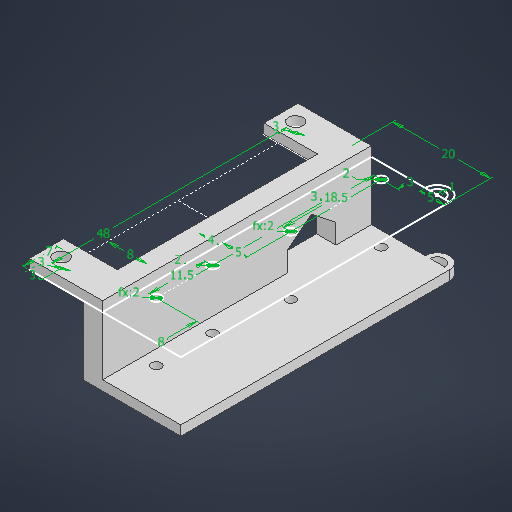
# Autodesk Inventor part: adcDAcmount
Saved by Autodesk Inventor 2025.1 (Build 291241000, 241)
## iProperties
Created: 2025-04-02
Part Number: adcDAcmount
Material: Generic
Document SubType Name: Modeling
Designer: jerem
Density: 1 g/cm^3
Appearance: Default
Author: jerem
## iProperties of the stored document adcDAcmount_3DPrint.ipt
Created: 2025-04-02
Part Number: adcDAcmount_3DPrint
Material: Generic
Document SubType Name: Modeling
Designer: jerem
Density: 1 g/cm^3
Appearance: Default
Author: jerem
Autodesk Inventor part; units mm, degrees
ref_plane "YZ Plane" through (0, 0, 0) normal (1, 0, 0) x (0, 1, 0)
ref_plane "XZ Plane" through (0, 0, 0) normal (0, 1, 0) x (-1, 0, 0)
ref_plane "XY Plane" through (0, 0, 0) normal (0, 0, 1) x (1, 0, 0)
sketch "Sketch1" plane through (0, 0, 0) normal (0, 1, 0) x (-1, 0, 0)
  line L0 (0, 0) -> (12, 0) construction
  line L1 (12, 24) -> (12, -24) construction
  circle A0 centre (12, 24) radius 1.5
  circle A1 centre (12, -24) radius 1.5
  line L2 (15, 27.5) -> (15, 20.5)
  line L3 (15, 20.5) -> (4, 20.5)
  line L4 (4, 20.5) -> (4, 0)
  line L5 (15, 27.5) -> (-16, 27.5)
  line L6 (4, 0) -> (12, 0) construction
  line L7 (15, -27.5) -> (15, -20.5)
  line L8 (15, -20.5) -> (4, -20.5)
  line L9 (4, -20.5) -> (4, 0)
  line L10 (15, -27.5) -> (-16, -27.5)
  line L11 (12, 24) -> (15, 24) construction
  line L12 (-16, 27.5) -> (-16, -27.5)
  line L13 (0, 27.5) -> (0, -27.5)
  line L14 (4, 20.5) -> (4, 27.5)
  line L15 (4, -20.5) -> (4, -27.5)
  circle A2 centre (-3, 8) radius 1
  circle A3 centre (-3, 19.5) radius 1
  line L16 (-3, 8) -> (-3, 19.5) construction
  circle A4 centre (-5, -24.5) radius 1
  circle A5 centre (-5, -6) radius 1
  line L17 (-5, -24.5) -> (-5, -6) construction
  arc A6 (-16, -27.5) -> (-11, -27.5) centre (-13.5, -27.5) ccw
  arc A7 (-15, -27.5) -> (-12, -27.5) centre (-13.5, -27.5) ccw
  point P0 (-12, -27.5)
  dimension "d0" = 3
  dimension "d1" = 3
  dimension "d2" = 3
  dimension "d3" = 7
  dimension "d4" = 48
  dimension "d5" = 8
  dimension "d7" = 4
  dimension "d12" = 20
  dimension "d13" = 2
  dimension "d14" = 2
  dimension "d15" = 11.5
  dimension "d16" = 3
  dimension "d17" = 2
  dimension "d18" = 2
  dimension "d19" = 18.5
  dimension "d20" = 5
  dimension "d23" = 8
  dimension "d24" = 3
  dimension "d27" = 5
  dimension "d28" = 1
  constraints: 36 end point, 8 centre point, 7 perpendicular, 6 point on line, 4 point on circle, 4 symmetric about line, 3 horizontal, 3 midpoint, 3 vertical, 2 coincident, 1 tangent
  measures "d0" diameter of A0
  measures "d1" diameter of A1
  measures "d2" distance of L11.start L11.end
  measures "d3" distance of L2.start L2.end
  measures "d4" distance of L1.start L1.end
  measures "d5" distance between parallel lines of L1 L4
  measures "d7" distance between parallel lines of L13 L4
  measures "d12" distance between parallel lines of L12 L15
  measures "d13" diameter of A2
  measures "d14" diameter of A3
  measures "d15" distance of L16.start L16.end
  measures "d16" distance between parallel lines of L13 L16
  measures "d17" diameter of A4
  measures "d18" diameter of A5
  measures "d19" distance of L17.start L17.end
  measures "d20" distance between parallel lines of L13 L17
  measures "d23" distance from line of L5 L16.end
  measures "d24" distance from line of L10 L17.start
  measures "d27" distance of L10.end A6.end
  measures "d28" radial gap between concentric circles of A6 A7
extrude "Extrusion1" add sketch "Sketch1" along normal blind 2 contours L2 L3 L14 L5 | L14 L4 L9 L15 L10 L13 L5 | L8 L7 L10 L15
extrude "Extrusion2" add sketch "Sketch1" against normal blind 14 contours L14 L4 L9 L15 L10 L13 L5
extrude "Extrusion3" add sketch "Sketch1" along normal blind 2 from surface at -14 contours L13 L10 L12 L5 | L10 A7 A6
sketch "Sketch2" plane through (0, 2, 27.5) normal (1, 0, 0) x (0, 0, -1)
  line L0 (55, -14) -> (0, -14) projected
  line L1 (55, -14) -> (55, 0) projected
  line L2 (0, 0) -> (55, 0) projected
  line L3 (0, -14) -> (0, 0) projected
  line L4 (32.5, -14) -> (34.5, -14) projected
  line L5 (51, -14) -> (53, -14) projected
  line L6 (33.5, -14) -> (52, -14)
  line L7 (42.75, -14) -> (42.75, -6) construction
  line L8 (42.75, -6) -> (37.75, -6)
  line L9 (37.75, -6) -> (37.75, -14)
  line L10 (42.75, -6) -> (47.75, -6)
  line L11 (47.75, -6) -> (47.75, -14)
  point P0 (27.5, -2)
  dimension "d29" = 10
  dimension "d30" = 8
  constraints: 12 end point, 3 midpoint, 3 perpendicular, 3 point on line, 1 collinear, 1 vertical
  measures "d29" distance of L8.end L10.end
  measures "d30" distance of L8.end L9.end
extrude "Extrusion4" cut sketch "Sketch2" against normal through all contours L0 L9 L8 L10 L11
chamfer "Chamfer1" distance 5 distance2 4 2 edges at (-2, -4, -10.25) (-2, -4, -20.25) measured on face at (-2.6667, -4, -13.5833)
equation "\"d14\" = d13"
equation "\"d18\" = d17"
body "Solid1"
